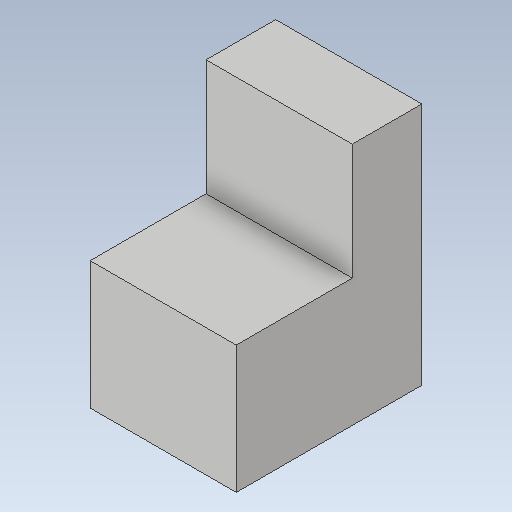
# Autodesk Inventor part: Fuel tank newest
Saved by Autodesk Inventor 2020 (Build 240168000, 168)
## iProperties
Created: 2020-10-15
Part Number: Fuel tank newest
Material: Generic
Document SubType Name: Modeling
Designer: nabee
Density: 1 g/cm^3
Appearance: Default
Mass: 23788.8 g
Surface Area: 5617.6 cm^2
Volume: 23788.8 cm^3
Author: nabee
Autodesk Inventor part; units mm, degrees
ref_plane "YZ Plane" through (0, 0, 0) normal (1, 0, 0) x (0, 1, 0)
ref_plane "XZ Plane" through (0, 0, 0) normal (0, 1, 0) x (-1, 0, 0)
ref_plane "XY Plane" through (0, 0, 0) normal (0, 0, 1) x (1, 0, 0)
sketch "Sketch2" plane through (0, 0, 0) normal (0, 0, 1) x (1, 0, 0)
  line L0 (0, 0) -> (180, 0)
  line L1 (180, 0) -> (180, 220)
  line L2 (180, 220) -> (0, 220)
  line L3 (0, 220) -> (0, 0)
  dimension "d4" = 220
  dimension "d5" = 180
  constraints: 8 end point, 2 parallel, 1 horizontal, 1 perpendicular
  measures "d4" distance of L0.end L1.end
  measures "d5" distance of L0.start L0.end
extrude "Extrusion2" add sketch "Sketch2" along normal blind 320
sketch "Sketch3" plane through (0, 220, 0) normal (0, 1, 0) x (1, 0, 0)
  line L0 (0, 0) -> (180, 0) projected
  line L1 (180, 0) -> (180, -320) projected
  line L2 (0, 0) -> (180, 0)
  line L3 (180, 0) -> (180, -120)
  line L4 (180, -120) -> (0, -120)
  line L5 (0, -120) -> (0, 0)
  dimension "d8" = 120
  constraints: 8 end point, 2 parallel, 1 horizontal, 1 perpendicular, 1 point on line
  measures "d8" distance of L4.end L0.start
extrude "Extrusion3" add sketch "Sketch3" along normal blind 200
sketch "Sketch4" plane through (0, 0, 0) normal (0, -1, 0) x (1, 0, 0)
  line L0 (0, 0) -> (180, 0) projected
  line L1 (180, 0) -> (180, 320) projected
  line L2 (0, 0) -> (180, 0)
  line L3 (180, 0) -> (180, 320)
  line L4 (180, 320) -> (0, 320)
  line L5 (0, 320) -> (0, 0)
  constraints: 8 end point, 2 parallel, 1 horizontal, 1 perpendicular
extrude "Extrusion4" add sketch "Sketch4" along normal blind 20
sketch "Sketch5" plane through (0, -20, 0) normal (0, -1, 0) x (1, 0, 0)
  line L0 (180, 320) -> (0, 320) projected
  line L1 (180, 120) -> (180, 0) projected
  line L2 (0, 320) -> (180, 320)
  line L3 (180, 320) -> (180, 0)
  line L4 (180, 0) -> (0, 0)
  line L5 (0, 0) -> (0, 320)
  constraints: 8 end point, 2 parallel, 1 horizontal, 1 perpendicular
extrude "Extrusion5" add sketch "Sketch5" along normal blind 40
sketch "Sketch6" plane through (180, 220, 120) normal (1, 0, 0) x (0, 0, -1)
  line L0 (0, 0) -> (-200, 0) projected
  line L1 (-200, 0) -> (0, 0)
  line L2 (120, 200) -> (0, 200) projected
  line L3 (0, 0) -> (0, 200)
  line L4 (0, 200) -> (120, 200)
  line L5 (120, 200) -> (120, -280) projected
  line L6 (120, 200) -> (120, -280)
  line L7 (120, -280) -> (-200, -280) projected
  line L8 (120, -280) -> (-200, -280)
  line L9 (-200, -280) -> (-200, 0)
  point P0 (120, -220)
  constraints: 12 end point, 4 perpendicular, 2 collinear
extrude "Extrusion6" add sketch "Sketch6" along normal blind 72
sketch "Sketch7" plane through (0, -60, 0) normal (0, -1, 0) x (1, 0, 0)
  line L0 (0, 0) -> (252, 0) projected
  line L1 (0, 320) -> (252, 320)
  line L2 (252, 320) -> (252, 0)
  line L3 (252, 0) -> (0, 0)
  line L4 (0, 0) -> (0, 320)
  constraints: 8 end point, 2 parallel, 1 horizontal, 1 perpendicular
extrude "Extrusion7" cut sketch "Sketch7" against normal blind 40
sketch "Sketch8" plane through (0, -20, 0) normal (0, -1, 0) x (1, 0, 0)
  line L0 (0, 120) -> (0, 320) projected
  line L1 (0, 0) -> (252, 0) projected
  line L2 (0, 320) -> (252, 320)
  line L3 (252, 320) -> (252, 0)
  line L4 (252, 0) -> (0, 0)
  line L5 (0, 0) -> (0, 320)
  constraints: 8 end point, 2 parallel, 1 horizontal, 1 perpendicular
extrude "Extrusion8" cut sketch "Sketch8" against normal blind 20
body "Solid2"
